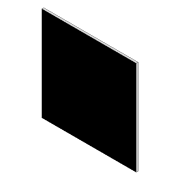
# Autodesk Inventor part: PCB Seguridad de Puertas
Saved by Autodesk Inventor 2020 (Build 240168000, 168)
## iProperties
Created: 2020-06-18
Part Number: PCB Seguridad de Puertas
Material: Generic
Document SubType Name: Modeling
Designer: Hernan
Density: 1 g/cm^3
Appearance: Default
Author: Hernan
Autodesk Inventor part; units mm, degrees
ref_plane "YZ Plane" through (0, 0, 0) normal (1, 0, 0) x (0, 1, 0)
ref_plane "XZ Plane" through (0, 0, 0) normal (0, 1, 0) x (-1, 0, 0)
ref_plane "XY Plane" through (0, 0, 0) normal (0, 0, 1) x (1, 0, 0)
sketch "Sketch1" plane through (0, 0, 0) normal (0, 0, 1) x (1, 0, 0)
  line L0 (-16.4515, -4.0205) -> (33.5485, -4.0205)
  line L1 (33.5485, -4.0205) -> (33.5485, 45.9795)
  line L2 (33.5485, 45.9795) -> (-16.4515, 45.9795)
  line L3 (-16.4515, 45.9795) -> (-16.4515, -4.0205)
  point P0 (0, 0)
  dimension "d0" = 50
  dimension "d1" = 50
  constraints: 8 end point, 3 perpendicular, 1 horizontal
  measures "d0" distance of L0.start L0.end
  measures "d1" distance of L0.end L1.end
extrude "Extrusion1" add sketch "Sketch1" along normal blind 1
body "Solid1"
